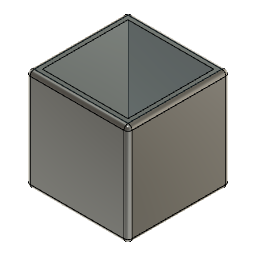
3D Print Test v1 (Autodesk Fusion 360 design; units mm, degrees)
Autodesk Fusion 360 part; units mm, degrees
sketch "Sketch1" plane through (0, 0, 0) normal (0, 0, 1) x (1, 0, 0)
  line L0 (-25, 0) -> (-25, -25)
  line L1 (-25, -25) -> (0, -25)
  line L2 (0, -25) -> (0, 0)
  line L3 (0, 0) -> (-25, 0)
  dimension "d1" = 25
  dimension "d2" = 25
  constraint vertical L0
  constraint perpendicular L0 L1
  constraint perpendicular L1 L2
  constraint perpendicular L0 L3
  measures "d1" distance of L1.end L2.end
  measures "d2" distance of L0.end L1.end
extrude "Extrude1" add sketch "Sketch1" along normal blind 25
fillet "Fillet1" radius 1 4 edges at (0, -12.5, 25) (0, -25, 12.5) (0, 0, 12.5) (0, -12.5, 0)
fillet "Fillet2" radius 1 11 edges at (-0.2929, -0.2929, 24.7071) (-13, 0, 25) (-25, -12.5, 25) (-13, -25, 25) (-0.2929, -24.7071, 24.7071) (-0.2929, -0.2929, 0.2929) (-13, 0, 0) (-25, -12.5, 0) (-25, -25, 12.5) (-13, -25, 0) (-0.2929, -24.7071, 0.2929)
fillet "Fillet3" radius 1 3 edges at (-24.7071, -0.2929, 0.2929) (-25, 0, 12.5) (-24.7071, -0.2929, 24.7071)
sketch "Sketch2" plane through (0, 0, 25) normal (0, 0, 1) x (-1, 0, 0)
  line L0 (1, 1) -> (24, 1)
  line L1 (24, 1) -> (24, 24)
  line L2 (24, 24) -> (1, 24)
  line L3 (1, 24) -> (1, 1)
shell "Shell2" thickness 2 removed faces 1 at (-8.6667, -8.6667, 25)
